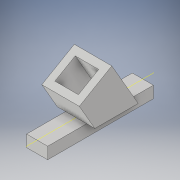
# Autodesk Inventor part: 60DegreeAttachementV02
Saved by Autodesk Inventor 2019.3 (Build 233278000, 278)
## iProperties
Created: 2019-02-16
Part Number: 60DegreeAttachementV02
Material: Generic
Document SubType Name: Modeling
Designer: steele
Density: 1 g/cm^3
Appearance: Default
Author: steele
Autodesk Inventor part; units mm, degrees
ref_plane "YZ Plane" through (0, 0, 0) normal (1, 0, 0) x (0, 1, 0)
ref_plane "XZ Plane" through (0, 0, 0) normal (0, 1, 0) x (-1, 0, 0)
ref_plane "XY Plane" through (0, 0, 0) normal (0, 0, 1) x (1, 0, 0)
sketch "Sketch1" plane through (0, 0, 0) normal (1, 0, 0) x (0, 1, 0)
  line L0 (0, 0) -> (29.1856, 16.8503)
  line L1 (29.1856, 16.8503) -> (49.5056, -18.345)
  line L2 (0, -73.2789) -> (0, 37.3579) projected
  line L3 (49.5056, -18.345) -> (0, -46.927)
  line L4 (0, 0) -> (0, -46.927)
  line L5 (32.9956, 10.2512) -> (0, -8.7988) construction
  dimension "d0" = 40.64
  dimension "d1" = 60
  dimension "d5" = 7.62
  dimension "d6" = 38.1
  constraints: 10 end point, 3 point on line, 2 parallel, 1 collinear, 1 perpendicular
  measures "d0" distance of L0.end L1.end
  measures "d1" angle of L0 L2
  measures "d5" distance between parallel lines of L5 L0
  measures "d6" distance from line of L5.end L1
extrude "Extrusion1" add sketch "Sketch1" along normal mid plane 40.64
sketch "Sketch2" plane through (-20.32, 29.1856, 16.8503) normal (0, 0.866, 0.5) x (1, 0, 0)
  line L0 (0, 0) -> (40.64, 0) construction
  line L1 (40.64, 0) -> (40.64, 40.64) construction
  line L2 (0, 0) -> (40.64, 40.64) construction
  line L3 (40.64, 40.64) -> (0, 40.64) construction
  line L4 (0, 40.64) -> (40.64, 0) construction
  line L5 (7.62, 7.62) -> (33.02, 7.62)
  line L6 (33.02, 7.62) -> (33.02, 33.02)
  line L7 (33.02, 33.02) -> (7.62, 33.02)
  line L8 (7.62, 33.02) -> (7.62, 7.62)
  line L9 (7.62, 7.62) -> (33.02, 33.02) construction
  line L10 (33.02, 7.62) -> (7.62, 33.02) construction
  point P0 (20.32, 0)
  point P1 (20.32, 20.32)
  dimension "d7" = 25.4
  constraints: 16 end point, 3 midpoint, 2 parallel, 2 perpendicular, 1 horizontal
  measures "d7" distance of L7.end L5.start
extrude "Extrusion2" cut sketch "Sketch2" against normal blind 38.1
sketch "Sketch3" plane through (0, 0, 0) normal (1, 0, 0) x (0, 1, 0)
  line L0 (29.1856, 16.8503) -> (0, 0) projected
  line L1 (0, 0) -> (0, -46.927) projected
  line L2 (0, -46.927) -> (49.5056, -18.345) projected
  line L3 (12.7, -30.7959) -> (0, -8.7988) projected
  line L4 (32.9956, 10.2512) -> (0, -8.7988) projected
  line L5 (0, 0) -> (0, -46.927)
  line L6 (29.1856, 16.8503) -> (15.6348, 16.8503) construction
  line L7 (0, 0) -> (29.1856, 16.8503) projected
  line L8 (0, 0) -> (0, 42.2503)
  line L9 (49.5056, -18.345) -> (0, -46.927) projected
  line L10 (0, -46.927) -> (0, -72.327)
  line L11 (0, -108.8389) -> (0, 72.9179) projected
  line L12 (0, 42.2503) -> (-12.7, 42.2503)
  line L13 (-12.7, 42.2503) -> (-12.7, -72.327)
  line L14 (-12.7, -72.327) -> (0, -72.327)
  point P0 (1.0999, -13.335)
  point P1 (0, -8.7988)
  dimension "d10" = 25.4
  dimension "d11" = 25.4
  dimension "d12" = 12.7
  constraints: 14 end point, 5 vertical, 2 horizontal, 2 perpendicular, 3 other
  measures "d10" distance from line of L8.end L6
  measures "d11" distance of L1.end L10.end
  measures "d12" distance of L8.end L12.end
extrude "Extrusion3" add sketch "Sketch3" along normal mid plane 22.86
equation "\"d0\" = widthToSupportExtrusion"
equation "\"d1\" = attachementAngle"
equation "\"d6\" = insertDepth"
equation "\"d2\" = widthToSupportExtrusion"
equation "\"d7\" = extrusionSize"
equation "\"d8\" = insertDepth"
equation "\"d12\" = supportBaseDepth"
equation "\"d13\" = supportBaseWidth"
equation "\"attachementAngle\" = 60deg"
equation "\"extrusionSize\" = 25.4"
equation "\"wallThickness\" = 6.35"
equation "\"slipClearance\" = 1.27"
equation "\"insertForExtrusion\" = extrusionSize + 2 * slipClearance"
equation "\"widthToSupportExtrusion\" = insertForExtrusion + 2 * wallThickness"
equation "\"insertDepth\" = 38.1"
equation "\"supportBaseWidth\" = 22.86"
equation "\"supportBaseDepth\" = 12.7"
body "Solid1"
